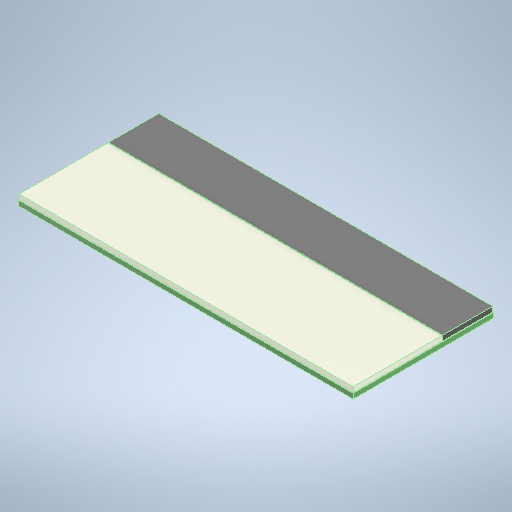
# Autodesk Inventor part: AQM1602XA
Saved by Autodesk Inventor 2025.3 (Build 293356000, 356)
## iProperties
Created: 2025-05-29
Part Number: AQM1602XA
Material: 一般
Document SubType Name: Modeling
Designer: yamashita1
Density: 1 g/cm^3
Appearance: 滑らか - 濃い深緑
Author: yamashita1
Autodesk Inventor part; units mm, degrees
ref_plane "YZ Plane" through (0, 0, 0) normal (1, 0, 0) x (0, 1, 0)
ref_plane "XZ Plane" through (0, 0, 0) normal (0, 1, 0) x (-1, 0, 0)
ref_plane "XY Plane" through (0, 0, 0) normal (0, 0, 1) x (1, 0, 0)
sketch "スケッチ1" plane through (0, 0, 0) normal (0, 0, 1) x (1, 0, 0)
  line L0 (-33, 27.7) -> (33, 27.7)
  line L1 (33, 27.7) -> (33, 0)
  line L2 (33, 0) -> (-33, 0)
  line L3 (-33, 0) -> (-33, 27.7)
  point P0 (0, 0)
  point P1 (0, 0)
  dimension "d0" = 66
  dimension "d1" = 27.7
  constraints: 8 end point, 2 parallel, 1 coincident, 1 horizontal, 1 midpoint, 1 perpendicular
  measures "d0" distance of L1.end L2.end
  measures "d1" distance of L0.end L1.end
extrude "押し出し1" add sketch "スケッチ1" along normal blind 1
sketch "スケッチ5" plane through (0, 0, 1) normal (0, 0, 1) x (1, 0, 0)
  line L0 (-32.9, 0.1) -> (32.9, 0.1)
  line L1 (32.9, 0.1) -> (32.9, 17.6)
  line L2 (32.9, 17.6) -> (-32.9, 17.6)
  line L3 (-32.9, 17.6) -> (-32.9, 0.1)
  line L4 (32.9, 17.7) -> (-32.9, 17.7)
  line L5 (-32.9, 17.7) -> (-32.9, 27.6)
  line L6 (-32.9, 27.6) -> (32.9, 27.6)
  line L7 (32.9, 27.6) -> (32.9, 17.7)
  line L8 (-33, 27.7) -> (-33, 0) projected
  line L9 (33, 27.7) -> (-33, 27.7) projected
  line L10 (33, 0) -> (33, 27.7) projected
  line L11 (-33, 0) -> (33, 0) projected
  point P0 (0, 0)
  dimension "d14" = 0.1
  dimension "d15" = 0.1
  dimension "d16" = 0.1
  dimension "d17" = 0.1
  dimension "d18" = 0.1
  dimension "d19" = 9.9
  constraints: 16 end point, 4 parallel, 2 horizontal, 2 perpendicular, 1 collinear, 1 point on line
  measures "d14" distance between parallel lines of L8 L5
  measures "d15" distance between parallel lines of L9 L6
  measures "d16" distance between parallel lines of L10 L7
  measures "d17" distance between parallel lines of L2 L4
  measures "d18" distance between parallel lines of L11 L0
  measures "d19" distance between parallel lines of L4 L6
extrude "押し出し4" add sketch "スケッチ5" along normal blind 1 contours L3 L2 L1 L0 | L4 L5 L6 L7
equation "\"d15\" = d14"
equation "\"d16\" = d14"
equation "\"d17\" = d14"
equation "\"d18\" = d14"
